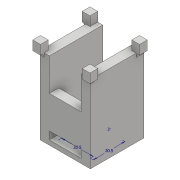
# Autodesk Inventor part: soft_gripper_base_1
Saved by Autodesk Inventor 2018 (Build 220112000, 112)
## iProperties
Created: 2018-07-20
Part Number: soft_gripper_base_1
Material: Generic
Document SubType Name: Sheet Metal
Designer: Bardo91
Density: 1 g/cm^3
Sheet Metal Rule: Default_mm
Appearance: Default
Author: Bardo91
Autodesk Inventor part; units mm, degrees
ref_plane "YZ Plane" through (0, 0, 0) normal (1, 0, 0) x (0, 1, 0)
ref_plane "XZ Plane" through (0, 0, 0) normal (0, 1, 0) x (-1, 0, 0)
ref_plane "XY Plane" through (0, 0, 0) normal (0, 0, 1) x (1, 0, 0)
sketch "Sketch1" plane through (0, 0, 0) normal (0, 0, 1) x (1, 0, 0)
  line L0 (0, 0) -> (20.5, 0)
  line L1 (20.5, 0) -> (20.5, 20.5)
  line L2 (20.5, 20.5) -> (0, 20.5)
  line L3 (0, 20.5) -> (0, 0)
  line L4 (-3, 23.5) -> (23.5, 23.5)
  line L5 (23.5, 23.5) -> (23.5, -3)
  line L6 (23.5, -3) -> (-3, -3)
  line L7 (-3, -3) -> (-3, 23.5)
  line L8 (0, 20.5) -> (0, 23.5)
  line L9 (20.5, 20.5) -> (20.5, 23.5)
  dimension "d0" = 20.5
  dimension "d1" = 20.5
  dimension "d2" = 3
  constraints: 20 end point, 6 perpendicular, 2 point on line, 1 horizontal, 1 parallel, 1 vertical, 3 other
  measures "d0" distance of L0.start L0.end
  measures "d1" distance of L0.end L1.end
  measures "d2" distance between parallel lines of L2 L4
extrude "Extrusion1" add sketch "Sketch1" along normal blind 3 contours L3 L2 L1 L0 | L8 L4 L9 L2
extrude "Extrusion2" add sketch "Sketch1" along normal blind 29 contours L0 L1 L9 L4 L5 L6 L7 L8 L3
sketch "Sketch2" plane through (0, 0, 3) normal (0, 1, 0) x (1, 0, 0)
  line L0 (0, 0) -> (20.5, 0)
  line L1 (20.5, 0) -> (20.5, -5)
  line L2 (20.5, -5) -> (0, -5)
  line L3 (0, -5) -> (0, 0)
  point P0 (0, 3)
  dimension "d7" = 20.5
  dimension "d8" = 5
  constraints: 8 end point, 2 parallel, 1 horizontal, 1 perpendicular
  measures "d7" distance of L1.end L2.end
  measures "d8" distance of L0.end L1.end
extrude "Extrusion3" cut sketch "Sketch2" against normal through all
sketch "Sketch4" plane through (-3, -3, 0) normal (0, -1, 0) x (1, 0, 0)
  line L0 (0, 0) -> (26.5, 0) projected
  line L1 (0, 0) -> (26.5, 0)
  line L2 (26.5, 0) -> (26.5, 29)
  line L3 (26.5, 29) -> (0, 29)
  line L4 (0, 29) -> (0, 0)
  line L5 (23.5, 3) -> (3, 3) projected
  line L6 (3, 8) -> (23.5, 8) projected
  line L7 (3, 3) -> (23.5, 3)
  line L8 (23.5, 3) -> (23.5, 8)
  line L9 (23.5, 8) -> (3, 8)
  line L10 (3, 8) -> (3, 3)
  point P0 (3, 0)
  constraints: 16 end point, 4 parallel, 2 horizontal, 2 perpendicular
extrude "Extrusion4" add sketch "Sketch4" along normal blind 3
sketch "Sketch5" plane through (0, 0, 29) normal (0, 0, 1) x (1, 0, 0)
  line L0 (-3, 23.5) -> (-3, -6) projected
  line L1 (0, 23.5) -> (-3, 23.5) projected
  line L2 (-3, -6) -> (0, -6)
  line L3 (0, -6) -> (0, 23.5)
  line L4 (0, 23.5) -> (-3, 23.5)
  line L5 (-3, 23.5) -> (-3, -6)
  line L6 (20.5, 23.5) -> (0, 23.5) projected
  line L7 (23.5424, -6) -> (20.5, -6)
  line L8 (20.5, -6) -> (20.5, 23.5)
  line L9 (20.5, 23.5) -> (23.5424, 23.5)
  line L10 (23.5424, 23.5) -> (23.5424, -6)
  point P0 (0, 0)
  constraints: 16 end point, 4 parallel, 2 horizontal, 2 perpendicular
extrude "Extrusion5" add sketch "Sketch5" along normal blind 21
sketch "Sketch6" plane through (-3, -6, 0) normal (0, -1, 0) x (1, 0, 0)
  line L0 (0, 0) -> (0, 50) projected
  line L1 (0, 0) -> (-3, 0)
  line L2 (-3, 0) -> (-3, 50)
  line L3 (-3, 50) -> (0, 50)
  line L4 (0, 50) -> (0, 0)
  line L5 (0, 0) -> (26.5, 0) projected
  line L6 (26.5, 0) -> (29.5, 0)
  line L7 (29.5, 0) -> (29.5, 50)
  line L8 (29.5, 50) -> (26.5, 50)
  line L9 (26.5, 50) -> (26.5, 0)
  point P0 (3, 0)
  dimension "d15" = 3
  dimension "d16" = 3
  constraints: 16 end point, 4 parallel, 2 horizontal, 2 perpendicular, 1 point on line
  measures "d15" distance of L2.end L3.end
  measures "d16" distance of L8.end L7.end
extrude "Extrusion6" add sketch "Sketch6" against normal up to surface (29.5 mm away)
sketch "Sketch8" plane through (0, 23.5, 3) normal (0, 1, 0) x (1, 0, 0)
  line L0 (-6, -47) -> (-6, 3) projected
  line L1 (-6, 3) -> (-6, -47)
  line L2 (-6, -47) -> (0, -47)
  line L3 (0, 0) -> (0, -47) projected
  line L4 (0, -47) -> (0, 0)
  line L5 (20.5, 0) -> (0, 0) projected
  line L6 (0, 0) -> (20.5, 0)
  line L7 (20.5, 0) -> (20.5, -47)
  line L8 (20.5, -47) -> (26.5, -47)
  line L9 (26.5, -47) -> (26.5, 3)
  line L10 (26.5, 3) -> (-6, 3)
  point P0 (0, 3)
  constraints: 16 end point, 5 perpendicular, 2 collinear, 2 point on line, 1 coincident
extrude "Extrusion7" add sketch "Sketch8" along normal blind 5
sketch "Sketch7" plane through (0, 0, 50) normal (0, 0, 1) x (1, 0, 0)
  line L0 (20.5, 0) -> (0, 0) projected
  line L1 (10.25, 0) -> (10.25, 10)
  line L2 (10.25, 10) -> (-3.25, 10)
  line L3 (-3.25, 10) -> (-3.25, -3.5)
  line L4 (-3.25, -3.5) -> (23.75, -3.5)
  line L5 (23.75, -3.5) -> (23.75, 23.5)
  line L6 (23.75, 23.5) -> (-3.25, 23.5)
  line L7 (-3.25, 23.5) -> (-3.25, 10)
  line L8 (-3.25, -3.5) -> (-8.25, -3.5)
  line L9 (-8.25, -3.5) -> (-8.25, -8.5)
  line L10 (-8.25, -8.5) -> (-3.25, -8.5)
  line L11 (-3.25, -8.5) -> (-3.25, -3.5)
  line L12 (-3.25, 23.5) -> (-8.25, 23.5)
  line L13 (-8.25, 23.5) -> (-8.25, 28.5)
  line L14 (-8.25, 28.5) -> (-3.25, 28.5)
  line L15 (-3.25, 28.5) -> (-3.25, 23.5)
  line L16 (23.75, 23.5) -> (28.75, 23.5)
  line L17 (28.75, 23.5) -> (28.75, 28.5)
  line L18 (28.75, 28.5) -> (23.75, 28.5)
  line L19 (23.75, 28.5) -> (23.75, 23.5)
  line L20 (23.75, -3.5) -> (28.75, -3.5)
  line L21 (28.75, -3.5) -> (28.75, -8.5)
  line L22 (28.75, -8.5) -> (23.75, -8.5)
  line L23 (23.75, -8.5) -> (23.75, -3.5)
  dimension "d19" = 10
  dimension "d20" = 13.5
  dimension "d21" = 13.5
  dimension "d22" = 27
  dimension "d23" = 27
  dimension "d24" = 27
  dimension "d25" = 5
  dimension "d26" = 5
  dimension "d27" = 5
  dimension "d28" = 5
  dimension "d29" = 5
  dimension "d30" = 5
  dimension "d31" = 5
  dimension "d32" = 5
  constraints: 46 end point, 8 parallel, 7 perpendicular, 6 horizontal, 1 midpoint, 1 vertical
  measures "d19" distance of L1.start L1.end
  measures "d20" distance of L1.end L2.end
  measures "d21" distance of L2.end L3.end
  measures "d22" distance of L3.end L4.end
  measures "d23" distance of L4.end L5.end
  measures "d24" distance of L5.end L6.end
  measures "d25" distance of L10.end L9.end
  measures "d26" distance of L9.end L8.end
  measures "d27" distance of L13.end L14.end
  measures "d28" distance of L12.end L13.end
  measures "d29" distance of L18.end L17.end
  measures "d30" distance of L17.end L16.end
  measures "d31" distance of L21.end L22.end
  measures "d32" distance of L20.end L21.end
extrude "Extrusion8" add sketch "Sketch7" along normal blind 6 contours L12 L13 L14 L15 | L19 L18 L17 L16 | L20 L21 L22 L23 | L11 L10 L9 L8
fillet "Fillet1" radius 2.5 6 edges at (26.5, 26, 50) (26.5, -4.75, 50) (25.125, -6, 50) (-4.625, -6, 50) (-6, -4.75, 50) (-6, 26, 50)
equation "\"BendRadius\" = Thickness"
equation "\"BendReliefWidth\" = Thickness"
equation "\"BendReliefDepth\" = 0.5 * Thickness"
equation "\"CornerReliefSize\" = 4 * Thickness"
equation "\"MinimumRemnant\" = 2 * Thickness"
equation "\"TransitionRadius\" = BendRadius"
equation "\"JacobiRadiusSize\" = BendRadius"
equation "\"GapSize\" = Thickness"
equation "\"Thickness\" = 0.5"
body "Solid1"
